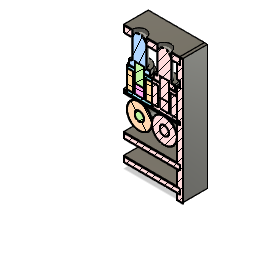
Braille Display Module CAD VA.1 (Autodesk Fusion 360 design; units mm, degrees)
Autodesk Fusion 360 part; units mm, degrees
note: some values were not read from the file. Chosen so that the rebuilt part matches the saved one: which bodies a step acts on; which face or edge a step refers to. Set by a fixed rule: which sketch regions a step uses.
sketch "Sketch1" plane through (0, 0, 0) normal (0, 0, 1) x (1, 0, 0)
  line L0 (-0.75, 2) -> (0.75, 2)
  line L1 (0.75, 2) -> (0.75, -2)
  line L2 (0.75, -2) -> (-0.75, -2)
  line L3 (-0.75, -2) -> (-0.75, 2)
  line L4 (0, 2) -> (0, -2)
  line L5 (0.75, -2) -> (2, -2)
  line L6 (2, -2) -> (2, -1.5)
  line L7 (2, -1.5) -> (0.75, -1.5)
  line L8 (0.75, -1.5) -> (0.75, -2)
  line L9 (0.75, -1.5) -> (-0.75, -1.5)
  line L10 (0.75, -1.5) -> (1, -1.5)
  line L11 (1, -1.5) -> (1, 2)
  line L12 (1, 2) -> (0.75, 2)
  line L13 (0.75, 2) -> (0.75, -1.5)
  line L14 (-0.75, -2) -> (-2, -2)
  line L15 (-2, -2) -> (-2, -1.5)
  line L16 (-2, -1.5) -> (-0.75, -1.5)
  line L17 (-0.75, -1.5) -> (-1, -1.5)
  line L18 (-1.25, 2.0006) -> (-0.75, 2)
  line L19 (-0.75, 2) -> (-0.75, -1.5)
  line L20 (-1, -1.5) -> (-1, 2)
  line L21 (1, 2) -> (2, 2)
  line L22 (2, 2) -> (2, 1.5)
  line L23 (2, 1.5) -> (1, 1.5)
  line L24 (1, 1.5) -> (1, 2)
  line L25 (2, -1.5) -> (2, 1.5)
  line L26 (-1, 2) -> (-2, 2)
  line L27 (-2, 2) -> (-2, 1.5)
  line L28 (-1, 1.5) -> (-1, 2)
  line L29 (-2, 1.5) -> (-1, 1.5)
  line L30 (-0.75, 0) -> (-0.75, 2.1)
  line L31 (-0.75, 2.1) -> (0.75, 2.1)
  line L32 (0.75, 2.1) -> (0.75, 0)
  line L33 (0, 2) -> (0, 2.1)
  line L34 (0.75, -1.5) -> (-0.75, -1.5)
  line L35 (-0.75, -1.5) -> (-0.75, 0)
  line L36 (-0.75, 0) -> (0.75, 0)
  line L37 (0.75, 0) -> (0.75, -1.5)
  line L38 (0.75, 2) -> (1.7, 2)
  line L39 (1.7, 2) -> (1.7, 2.1)
  line L40 (1.7, 2.1) -> (0.75, 2.1)
  line L41 (0.75, 2.1) -> (0.75, 2)
  line L42 (0.75, 2.1) -> (-0.75, 2.1)
  line L43 (-0.75, 2.1) -> (-0.75, 3)
  line L44 (-0.75, 3) -> (0.75, 3)
  line L45 (0.75, 3) -> (0.75, 2.1)
  line L46 (1.125, 2.1) -> (1.125, 3)
  line L47 (1.125, 3) -> (0.75, 3)
  line L48 (0, 3) -> (0, 4.8844)
  line L49 (0, 2.1) -> (0, 7.15)
  line L50 (1.125, 3) -> (1.125, 7.15)
  line L51 (1.125, 7.15) -> (-0.75, 7.15)
  line L52 (-0.75, 7.15) -> (-0.75, 3)
  line L53 (-1.125, 2.1) -> (-1.125, 3)
  line L54 (-1.125, 3) -> (-1.125, 7.15)
  line L55 (0.75, 7.15) -> (0.75, 3)
  line L56 (-0.75, 7.15) -> (-1.125, 7.15)
  line L57 (-0.75, 3) -> (-1.125, 3)
  line L58 (-0.75, 2.1) -> (-1.125, 2.1)
  line L59 (-1.125, 2.1) -> (-1.8, 2.1)
  line L60 (-1.8, 2.1) -> (-1.8, 2)
  line L61 (-1.125, 7.15) -> (-3, 7.15)
  line L62 (-3, 7.15) -> (-3, 6.15)
  line L63 (-3, 6.15) -> (-1.125, 6.15)
  line L64 (-1.125, 6.15) -> (-1.125, 7.15)
  line L65 (-3, 6.15) -> (-2, 6.15)
  line L66 (-2, 6.15) -> (-2, -2)
  line L67 (-2, -2) -> (-3, -2)
  line L68 (-3, -2) -> (-3, 6.15)
  line L69 (4.75, 2) -> (4.75, -1.5)
  line L70 (3.25, 2) -> (3.25, -1.5)
  line L71 (4.75, -2) -> (4.75, 2)
  line L72 (2, 1.5) -> (3, 1.5)
  line L73 (5, -1.5) -> (5, 2)
  line L74 (3, -1.5) -> (3, 2)
  line L75 (4, 2) -> (4, -2)
  line L76 (3.25, -2) -> (2, -2)
  line L77 (4.75, 2.1) -> (5.125, 2.1)
  line L78 (3.25, 2) -> (2.3, 2)
  line L79 (4.75, -2) -> (6, -2)
  line L80 (3.25, 0) -> (3.25, -1.5)
  line L81 (3.25, -1.5) -> (4.75, -1.5)
  line L82 (3.25, -1.5) -> (3, -1.5)
  line L83 (6, -2) -> (6, -1.5)
  line L84 (5.125, 2.1) -> (5.8, 2.1)
  line L85 (2.3, 2) -> (2.3, 2.1)
  line L86 (6, -1.5) -> (4.75, -1.5)
  line L87 (6, 6.15) -> (6, -2)
  line L88 (4.75, 3) -> (5.125, 3)
  line L89 (4, 3) -> (4, 4.8844)
  line L90 (3.25, 3) -> (3.25, 2.1)
  line L91 (7, -2) -> (7, 6.15)
  line L92 (3.25, -1.5) -> (4.75, -1.5)
  line L93 (4, 2.1) -> (4, 7.15)
  line L94 (3.25, 7.15) -> (3.25, 3)
  line L95 (6, 1.5) -> (5, 1.5)
  line L96 (4.75, -1.5) -> (4.75, 0)
  line L97 (2, -1.5) -> (3.25, -1.5)
  line L98 (4.75, -1.5) -> (5, -1.5)
  line L99 (3.25, 2) -> (3.25, -2)
  line L100 (5.125, 3) -> (5.125, 7.15)
  line L101 (4.75, 7.15) -> (4.75, 3)
  line L102 (4.75, 3) -> (3.25, 3)
  line L103 (2.875, 3) -> (2.875, 7.15)
  line L104 (2.3, 2.1) -> (3.25, 2.1)
  line L105 (5.125, 7.15) -> (7, 7.15)
  line L106 (3.25, -2) -> (4.75, -2)
  line L107 (3.25, -1.5) -> (3.25, -2)
  line L108 (4.75, 0) -> (3.25, 0)
  line L109 (3, 1.5) -> (3, 2)
  line L110 (7, 6.15) -> (6, 6.15)
  line L111 (2.875, 2.1) -> (2.875, 3)
  line L112 (6, -2) -> (7, -2)
  line L113 (3.25, 2.1) -> (3.25, 2)
  line L114 (7, 6.15) -> (5.125, 6.15)
  line L115 (4.75, 2) -> (3.25, 2)
  line L116 (5, 2) -> (6, 2)
  line L117 (4, 2) -> (4, 2.1)
  line L118 (3, 2) -> (2, 2)
  line L119 (5, 1.5) -> (5, 2)
  line L120 (7, 7.15) -> (7, 6.15)
  line L121 (4.75, 7.15) -> (5.125, 7.15)
  line L122 (4.75, 0) -> (4.75, 2.1)
  line L123 (4.75, 2.1) -> (3.25, 2.1)
  line L124 (5, 2) -> (4.75, 2)
  line L125 (3, 2) -> (3.25, 2)
  line L126 (2.875, 3) -> (3.25, 3)
  line L127 (5.125, 6.15) -> (5.125, 7.15)
  line L128 (5.8, 2.1) -> (5.8, 2)
  line L129 (2.875, 7.15) -> (4.75, 7.15)
  line L130 (6, 2) -> (6, 1.5)
  line L131 (4.75, 2.1) -> (4.75, 3)
  line L132 (3.25, 2.1) -> (4.75, 2.1)
  line L133 (3.25, 2.1) -> (3.25, 0)
  line L134 (5.125, 2.1) -> (5.125, 3)
  line L135 (1.125, 7.15) -> (2.875, 7.15)
  line L136 (2.875, 7.15) -> (2.875, 6.15)
  line L137 (2.875, 6.15) -> (1.125, 6.15)
  line L138 (1.125, 6.15) -> (1.125, 7.15)
  line L139 (5.125, 6.15) -> (-1.125, 6.15)
  line L140 (-1.125, 6.15) -> (-1.125, 7.15)
  line L141 (-1.125, 7.15) -> (5.125, 7.15)
  line L142 (5.125, 7.15) -> (5.125, 6.15)
  line L143 (-3, -2) -> (7, -2)
  line L144 (7, -2) -> (7, -2.25)
  line L145 (7, -2.25) -> (-3, -2.25)
  line L146 (-3, -2.25) -> (-3, -2)
  arc A0 (5.125, 6.15) -> (2.875, 6.15) centre (4, 6.0172) ccw
  arc A1 (1.125, 6.15) -> (-1.125, 6.15) centre (0, 6.0172) ccw
  line L147 (-2.5, 2.9) -> (-2.5, 3.9)
  line L148 (-2.5, 3.9) -> (-2, 3.9)
  line L149 (-2, 2.9) -> (-2.5, 2.9)
  line L150 (6, 2.9) -> (6.5, 2.9)
  line L151 (6.5, 2.9) -> (6.5, 3.9)
  line L152 (6.5, 3.9) -> (6, 3.9)
  line L153 (1.7, 2.1) -> (-1.8, 2.1)
  line L154 (-1.8, 2.1) -> (-1.8, 2.85)
  line L155 (-1.8, 2.85) -> (1.7, 2.85)
  line L156 (1.7, 2.85) -> (1.7, 2.1)
  line L157 (2.3, 2.1) -> (5.8, 2.1)
  line L158 (5.8, 2.1) -> (5.8, 2.85)
  line L159 (2.3, 2.85) -> (2.3, 2.1)
  line L160 (5.8, 2.85) -> (2.3, 2.85)
  line L161 (7, -1.75) -> (-3, -1.75)
  line L162 (6, -1.75) -> (6.5, -1.75)
  line L163 (6.5, -1.75) -> (6.5, -2.25)
  line L164 (6.5, -2.25) -> (6, -2.25)
  line L165 (6, -2.25) -> (6, -1.75)
  line L166 (-3, 7.15) -> (-2.5, 7.15)
  line L167 (-2.5, 7.15) -> (-2.5, 6.15)
  line L168 (-2.5, 6.15) -> (-3, 6.15)
  line L169 (-3, 6.15) -> (-3, 7.15)
  line L170 (7, 7.15) -> (6.5, 7.15)
  line L171 (6.5, 6.15) -> (7, 6.15)
  line L172 (7, 6.15) -> (7, 7.15)
  line L173 (6.5, 7.15) -> (6.5, 6.15)
  line L174 (-2, -2.25) -> (-2, -1.75)
  line L175 (-2, -1.75) -> (-2.5, -1.75)
  line L176 (-2.5, -2.25) -> (-2, -2.25)
  line L177 (-2.5, -1.75) -> (-2.5, -2.25)
  line L178 (-3, -2.25) -> (-2, -2.25)
  line L179 (-2, -2.25) -> (-2, -12.85)
  line L180 (-2, -12.85) -> (-3, -12.85)
  line L181 (-3, -12.85) -> (-3, -2.25)
  line L182 (7, -2.25) -> (6, -2.25)
  line L183 (6, -2.25) -> (6, -12.85)
  line L184 (6, -12.85) -> (7, -12.85)
  line L185 (7, -12.85) -> (7, -2.25)
  line L186 (-2.5, -7.75) -> (6.5, -7.75)
  line L187 (6.5, -7.75) -> (6.5, -8.55)
  line L188 (6.5, -8.55) -> (-2.5, -8.55)
  line L189 (-2.5, -8.55) -> (-2.5, -7.75)
  line L190 (-2.5, -11.05) -> (6.5, -11.05)
  line L191 (6.5, -11.05) -> (6.5, -11.85)
  line L192 (6.5, -11.85) -> (-2.5, -11.85)
  line L193 (-2.5, -11.85) -> (-2.5, -11.05)
  line L194 (-2, -6.25) -> (6, -6.25)
  line L195 (2, -2.25) -> (2, -6.25)
  line L196 (2, -4.25) -> (6, -4.25) construction
  circle A2 centre (0, -4.25) radius 0.75
  circle A3 centre (4, -4.25) radius 0.75
  circle A4 centre (0, -4.25) radius 2
  circle A5 centre (4, -4.25) radius 2
  point P0 (4, 0)
  dimension "d4" = 0.25
  dimension "d7" = 0.5
  dimension "d8" = 4
  dimension "d9" = 0.5
  dimension "d21" = 1.5
  dimension "d22" = 1.5
  dimension "d27" = 0.1
  dimension "d31" = 1
  dimension "d32" = 1
  dimension "d37" = 0.25
  dimension "d57" = 1
  dimension "d60" = 0.5
  dimension "d63" = 1.8
  dimension "d64" = 0.75
  dimension "d68" = 2.25
  dimension "d69" = 3
  dimension "d70" = 3
  dimension "d72" = 2.25
  dimension "d73" = 0.25
  dimension "d74" = 0.5
  dimension "d76" = 0.5
  dimension "d77" = 0.5
  dimension "d78" = 0.8
  dimension "d79" = 0.8
  dimension "d80" = 0.5
  dimension "d81" = 0.5
  dimension "d82" = 2.5
  dimension "d85" = 1.5
  dimension "d97" = 4
  dimension "d100" = 1.5
  dimension "d101" = 1.5
  dimension "d104" = 3.5
  dimension "d105" = 20
  constraint horizontal L0
  constraint vertical L1
  constraint horizontal L2
  constraint vertical L3
  constraint midpoint L0 L4.start
  constraint midpoint L2 L4.end
  constraint coincident origin L4
  constraint horizontal L5
  constraint vertical L6
  constraint horizontal L7
  constraint vertical L8
  constraint coincident L3 L9.end
  constraint perpendicular L3 L9
  constraint horizontal L10
  constraint vertical L11
  constraint horizontal L12
  constraint vertical L13
  constraint coincident L0.end L1.start
  constraint symmetric L1.end L4 L2.end
  constraint symmetric L4 L5.end L14.end
  constraint symmetric L4 L6.end L15.end
  constraint symmetric L4 L7.end L9.end
  constraint symmetric L4 L10.end L17.end
  constraint symmetric L4 L11.end L20.end
  constraint symmetric L4 L0.end L0.start
  constraint horizontal L21
  constraint vertical L22
  constraint horizontal L23
  constraint vertical L24
  constraint vertical L25
  constraint symmetric L4 L21.end L26.end
  constraint symmetric L4 L22.end L27.end
  constraint symmetric L4 L23.end L28.start
  constraint vertical L30
  constraint horizontal L31
  constraint vertical L32
  constraint perpendicular L31 L33
  constraint coincident L31 L33.end
  constraint horizontal L34
  constraint vertical L35
  constraint horizontal L36
  constraint vertical L37
  constraint coincident L19 L30.start
  constraint coincident L3 L30.start
  constraint coincident L1 L32.end
  constraint coincident L32.end L36.end
  constraint coincident L30.start L36
  constraint coincident origin L36
  constraint horizontal L38
  constraint vertical L39
  constraint horizontal L40
  constraint vertical L41
  constraint coincident L32 L0.end
  constraint coincident L21 L38.end
  constraint horizontal L42
  constraint vertical L43
  constraint horizontal L44
  constraint vertical L45
  constraint coincident L30.end L31.start
  constraint coincident L31.end L32.start
  constraint coincident L40 L46.start
  constraint perpendicular L40 L46
  constraint horizontal L47
  constraint midpoint L44 L48.start
  constraint perpendicular L44 L48
  constraint perpendicular L43 L51
  constraint perpendicular L44 L52
  constraint symmetric L46.end L48 L53.end
  constraint symmetric L43.end L48 L44.end
  constraint symmetric L46.start L48 L53.start
  constraint symmetric L48 L50.end L54.end
  constraint symmetric L48 L51.end L55.start
  constraint perpendicular L43 L59
  constraint coincident L26 L60.end
  constraint perpendicular L26 L60
  constraint horizontal L61
  constraint vertical L62
  constraint horizontal L63
  constraint vertical L64
  constraint horizontal L65
  constraint vertical L66
  constraint horizontal L67
  constraint vertical L68
  constraint symmetric origin L25 P0
  constraint symmetric L0.start L25 L69.start
  constraint symmetric L0.end L25 L70.start
  constraint symmetric L1.end L25 L76.start
  constraint symmetric L2.end L25 L71.start
  constraint symmetric L4.start L25 L75.start
  constraint symmetric L4.end L25 L75.end
  constraint symmetric L32.end L25 L80.start
  constraint symmetric L5.end L25 L6.start
  constraint symmetric L6.end L25 L7.start
  constraint symmetric L7.end L25 L70.end
  constraint symmetric L9.end L25 L69.end
  constraint symmetric L10.end L25 L74.start
  constraint symmetric L11.end L25 L74.end
  constraint symmetric L14.end L25 L79.end
  constraint symmetric L15.end L25 L83.end
  constraint symmetric L17.end L25 L73.start
  constraint symmetric L20.end L25 L73.end
  constraint symmetric L21.end L25 L22.start
  constraint symmetric L22.end L25 L23.start
  constraint symmetric L23.end L25 L72.end
  constraint symmetric L25 L20.end L73.end
  constraint symmetric L25 L26.end L116.end
  constraint symmetric L25 L27.end L95.start
  constraint symmetric L25 L28.start L95.end
  constraint symmetric L25 L30.start L96.end
  constraint symmetric L25 L30.end L77.start
  constraint symmetric L25 L31.end L90.end
  constraint symmetric L25 L33.end L93.start
  constraint symmetric L25 L9.end L69.end
  constraint symmetric L25 L32.end L80.start
  constraint symmetric L25 L0.end L70.start
  constraint symmetric L25 L38.end L78.end
  constraint symmetric L25 L39.end L85.end
  constraint symmetric L25 L43.end L88.start
  constraint symmetric L25 L44.end L90.start
  constraint symmetric L25 L46.start L111.start
  constraint symmetric L25 L46.end L103.start
  constraint symmetric L25 L48.start L89.start
  constraint symmetric L25 L48.end L89.end
  constraint symmetric L25 L49.end L93.end
  constraint symmetric L25 L50.end L103.end
  constraint symmetric L25 L51.end L101.start
  constraint symmetric L25 L53.end L88.end
  constraint symmetric L25 L53.start L77.end
  constraint symmetric L25 L54.end L100.end
  constraint symmetric L25 L55.start L94.start
  constraint symmetric L25 L59.end L84.end
  constraint symmetric L25 L60.end L128.end
  constraint symmetric L25 L61.end L105.end
  constraint symmetric L25 L62.end L91.end
  constraint symmetric L25 L63.end L114.end
  constraint symmetric L25 L65.end L87.start
  constraint symmetric L25 L67.end L91.start
  constraint horizontal L135
  constraint vertical L136
  constraint horizontal L137
  constraint vertical L138
  constraint coincident L103 L136.end
  constraint horizontal L139
  constraint vertical L140
  constraint horizontal L141
  constraint vertical L142
  constraint horizontal L143
  constraint vertical L144
  constraint horizontal L145
  constraint vertical L146
  constraint coincident L91.start L112.end
  constraint coincident L89.end A0
  constraint tangent L141 A0
  constraint symmetric L25 L114.end L63.end
  constraint symmetric L25 L136.end L137.end
  constraint symmetric L25 A0 A1
  constraint coincident L139 L114.end
  constraint vertical L100
  constraint coincident L114.end L127.start
  constraint coincident L136.end L137.start
  constraint perpendicular L26 L147
  constraint coincident L66 L148.end
  constraint perpendicular L66 L148
  constraint coincident L66 L149.start
  constraint horizontal L149
  constraint horizontal L26
  constraint coincident L26.end L27.start
  constraint symmetric L25 L147.start L150.end
  constraint symmetric L25 L147.end L151.end
  constraint symmetric L25 L148.end L152.end
  constraint symmetric L25 L149.start L150.start
  constraint horizontal L153
  constraint vertical L154
  constraint horizontal L155
  constraint vertical L156
  constraint coincident L59.end L60.start
  constraint symmetric L25 L154.end L158.end
  constraint symmetric L25 L155.end L159.start
  constraint coincident L139 L137.end
  constraint coincident L91 L161.start
  constraint coincident L68 L161.end
  constraint perpendicular L68 L161
  constraint horizontal L162
  constraint vertical L163
  constraint horizontal L164
  constraint vertical L165
  constraint coincident L145 L163.end
  constraint midpoint L83 L162.start
  constraint horizontal L166
  constraint vertical L167
  constraint horizontal L168
  constraint vertical L169
  constraint midpoint L65 L167.end
  constraint symmetric L25 L162.start L174.end
  constraint symmetric L25 L162.end L175.end
  constraint symmetric L25 L163.end L176.start
  constraint symmetric L25 L164.end L174.start
  constraint symmetric L25 L166.end L170.end
  constraint symmetric L25 L167.end L171.start
  constraint horizontal L178
  constraint vertical L179
  constraint horizontal L180
  constraint vertical L181
  constraint coincident L174.start L176.end
  constraint horizontal L182
  constraint vertical L183
  constraint horizontal L184
  constraint vertical L185
  constraint coincident L164.end L165.start
  constraint equal L179 L183
  constraint horizontal L186
  constraint vertical L187
  constraint horizontal L188
  constraint vertical L189
  constraint horizontal L190
  constraint vertical L191
  constraint horizontal L192
  constraint vertical L193
  constraint coincident L179 L194.start
  constraint coincident L183 L194.end
  constraint perpendicular L183 L194
  constraint coincident L49.end L141
  constraint midpoint L145 L195.start
  constraint midpoint L194 L195.end
  constraint midpoint L195 L196.start
  constraint coincident L183 L196.end
  constraint perpendicular L183 L196
  constraint concentric A2 A4
  constraint tangent L194 A4
  constraint concentric A3 A5
  constraint tangent L194 A5
  constraint tangent L195 A5
  constraint tangent L195 A4
  constraint tangent L145 A4
  constraint tangent L145 A5
  measures "d4" distance of L11.end L0.end
  measures "d7" distance of L5 L7
  measures "d8" distance of L5.end L14.end
  measures "d9" distance of L21 L23
  measures "d21" distance of L30.end L31.end
  measures "d22" distance of L9 L36
  measures "d27" distance of L38.end L39.end
  measures "d31" distance of L66 L68
  measures "d32" distance of L61 L63
  measures "d37" distance of L112 L145
  measures "d57" distance of L147.start L147.end
  measures "d60" distance of L66 L147
  measures "d63" vertical distance of L59.end L147.end
  measures "d64" distance of L153 L155
  measures "d68" distance of L46 L53
  measures "d69" distance of L36 L44
  measures "d70" distance of L16 L29
  measures "d72" distance of L65 L148
  measures "d73" distance of L143 L161
  measures "d74" distance of L163 L165
  measures "d76" distance of L179 L189
  measures "d77" distance of L183 L187
  measures "d78" distance of L186 L188
  measures "d79" distance of L190 L192
  measures "d80" distance of L183 L191
  measures "d81" distance of L179 L193
  measures "d82" distance of L188 L190
  measures "d85" distance of L186 L194
  measures "d97" distance of L145 L194
  measures "d100" diameter of A2
  measures "d101" diameter of A3
  measures "d104" distance of L154 L156
  measures "d105" distance of L61.end L180
revolve "Revolve1" add sketch "Sketch1" angle 360 about axis through (0, 1.75, 0) along (0, 1, 0) contours L1 L7 L10 L11 L12 L13 L24 L32 L37 L38 | L11 L21 L22 L23 L24 L38 | L1 L4 L8 L9 L34 L161 | L1 L6 L7 L8 L10 L161 | L1 L2 L4 L8 L143 L161 | L1 L5 L6 L8 L143 L161 makes body 1
revolve "Revolve2" add sketch "Sketch1" angle 360 about axis through (0, 1.75, 0) along (0, 1, 0) separate body contours L1 L4 L9 L13 L34 L36 L37 makes body 2
revolve "Revolve3" add sketch "Sketch1" angle 360 about axis through (0, 1.75, 0) along (0, 1, 0) separate body contours L7 L11 L23 L25 makes body 3
revolve "Revolve4" add sketch "Sketch1" angle 360 about axis through (0, 2, 0) along (0, 1, 0) separate body contours L0 L31 L32 L33 L41 L42 L153 | L0 L1 L4 L13 L32 L36 | L31 L42 L45 L49 L153 L155 | L44 L45 L49 L155 makes body 4
revolve "Revolve5" add sketch "Sketch1" angle 360 about axis through (0, 2.1, 0) along (0, 1, 0) separate body contours L40 L45 L46 L153 L155 | L40 L46 L153 L155 L156 | L45 L46 L47 L155 | L44 L48 L49 L55 L139 | L47 L50 L55 L139 | L49 L55 L139 A1 | L55 L139 A1 makes body 5
revolve "Revolve7" add sketch "Sketch1" angle 360 about axis through (0, 2, 0) along (0, -1, 0) separate body contours L12 L21 L32 L38 L39 L40 L41 L153 makes body 6
extrude "Extrude1" add sketch "Sketch1" along normal blind 12 and the other way blind 4 separate body contours L15 L27 L63 L65 L66 L68 L147 L148 L149 L161 L168 L175 | L67 L68 L143 L161 L177 | L67 L143 L145 L146 L177 L178 | L145 L176 L178 L179 L180 L181 L186 L188 L189 L190 L192 L193 | L61 L62 L63 L65 L166 L167 L168 L169 | L83 L87 L91 L110 L114 L130 L150 L151 L152 L161 L162 L171 | L145 L164 L182 L183 L184 L185 L186 L187 L188 L190 L191 L192 | L91 L112 L143 L161 L163 | L112 L143 L144 L145 L163 L182 | L105 L110 L114 L120 L170 L171 L172 L173 makes body 7 at (-3, -6.1833, 6.6667) makes body 8 at (7, 0.4833, 1.3333)
extrude "Extrude4" add sketch "Sketch1" along normal blind 12 and the other way blind 4 separate body contours L2 L3 L4 L143 L161 | L3 L14 L15 L66 L143 L161 L174 | L1 L2 L4 L8 L143 L161 | L15 L66 L67 L143 L161 L174 L175 L177 | L52 L139 A1 | L49 L52 L139 A1 | L1 L5 L6 L8 L143 L161 | L52 L54 L56 L64 L140 L141 A1 | L51 L52 L141 A1 | L49 L55 L139 A1 | L54 L61 L63 L64 L65 L140 L167 | L6 L76 L99 L107 L143 L161 | L55 L139 A1 | L51 L55 L141 A1 | L75 L99 L106 L107 L143 L161 | L50 L51 L55 L138 L141 A1 | L50 L103 L135 L136 L137 L138 L139 L141 | L71 L75 L106 L143 L161 | L94 L139 A0 | L94 L103 L129 L136 L141 A0 | L71 L79 L83 L87 L143 L161 L165 | L93 L94 L139 A0 | L94 L129 L141 A0 | L179 L183 L186 L188 | L179 L186 L188 L189 | L83 L87 L112 L143 L161 L162 L163 L165 | L93 L101 L139 A0 | L101 L129 L141 A0 | L183 L186 L187 L188 | L101 L139 A0 | L100 L101 L121 L127 L141 L142 A0 | L179 L190 L192 L193 | L179 L183 L190 L192 | L100 L105 L110 L114 L127 L142 L173 | L183 L190 L191 L192 makes body 9 at (3.5, -2, 6.6667) makes body 10 at (0.5, -7.75, 6.6667) makes body 11 at (3.5, 6.15, 1.3333) makes body 12 at (0.5, -11.05, 6.6667)
extrude "Extrude5" add sketch "Sketch1" along normal blind 12 and the other way blind 4 separate body contours L2 L5 L14 L76 L79 L106 L143 L145 L165 L174 | L67 L143 L145 L174 L176 L177 L178 | L112 L143 L145 L163 L164 L165 L182 makes body 13
revolve "Revolve6" cut sketch "Sketch1" angle 360 about axis through (0, 3, 0) along (0, 1, 0) contours L1 L2 L4 L8 L143 L161 | L44 L48 L49 L55 L139 | L1 L5 L6 L8 L143 L161 | L47 L50 L55 L139 | L49 L55 L139 A1 | L55 L139 A1 | L51 L55 L141 A1 | L50 L51 L55 L138 L141 A1 bodies 9 11
pattern_linear "R-Pattern2" count 2 spacing 4 along (1, 0, 0) count 3 spacing 4 along (0, 0, 1) of "Revolve6"
pattern_linear "R-Pattern1" count 2 spacing 4 along (1, 0, 0) count 3 spacing 4 along (0, 0, 1) of bodies 5 3 1 4 2 6 makes body 14 at (5.5759, -2, 0.0994) makes body 15 at (1.5759, -2, 4.0994) makes body 16 at (5.5759, -2, 4.0994) makes body 17 at (1.5759, -2, 8.0994) makes body 18 at (5.5759, -2, 8.0994) makes body 19 at (4.7491, -0.5, 0.0374) makes body 20 at (0.7491, -0.5, 4.0374) makes body 21 at (4.7491, -0.5, 4.0374) makes body 22 at (0.7491, -0.5, 8.0374) makes body 23 at (4.7491, -0.5, 8.0374) makes body 24 at (5.9901, -0.5, 0.1991) makes body 25 at (1.9901, -0.5, 4.1991) makes body 26 at (5.9901, -0.5, 4.1991) makes body 27 at (1.9901, -0.5, 8.1991) makes body 28 at (5.9901, -0.5, 8.1991) makes body 29 at (4.7491, 1.3333, 0.0374) makes body 30 at (0.7491, 1.3333, 4.0374) makes body 31 at (4.7491, 1.3333, 4.0374) makes body 32 at (-0.7463, 1.3333, 8.0747) makes body 33 at (3.2537, 1.3333, 8.0747) makes body 34 at (5.1236, 4.05, 0.0561) makes body 35 at (1.1236, 4.05, 4.0561) makes body 36 at (5.1236, 4.05, 4.0561) makes body 37 at (1.1236, 4.05, 8.0561) makes body 38 at (5.1236, 4.05, 8.0561) makes body 39 at (5.6916, 2.0667, -0.1693) makes body 40 at (1.6979, 2.0333, 3.9153) makes body 41 at (5.6916, 2.0667, 3.8307) makes body 42 at (1.6979, 2.0333, 7.9153) makes body 43 at (5.6916, 2.0667, 7.8307)
extrude "Extrude6" cut 2 faces at (1.9044, -1.75, 6.1628) (1.9044, -1.75, 2.1628) along direction (0, -1, 0) blind 1 on bodies 9 bodies 9
extrude "Extrude7" add sketch "Sketch1" along normal blind 12 and the other way blind 4 separate body contours A5 | A2 makes body 44 at (0.7491, -4.2874, 8) makes body 45 at (5.9901, -4.4491, 1.3333)
extrude "Extrude8" add sketch "Sketch1" along normal blind 12 and the other way blind 4 separate body contours A4 | A3 makes body 46 at (1.9901, -4.4491, 1.3333) makes body 47 at (4.7491, -4.2874, 8)
copy_body "Body->Comp1" bodies 1 removing the originals makes body 48 in component "Magnet Core"
copy_body "Body->Comp2" bodies 2 removing the originals makes body 49 in component "Magnet"
copy_body "Body->Comp3" bodies 3 removing the originals makes body 50 in component "Coil"
copy_body "Body->Comp4" bodies 4 removing the originals makes body 51 in component "Pin"
copy_body "Body->Comp5" bodies 5 removing the originals makes body 52 in component "PinHat"
copy_body "Body->Comp6" bodies 6 removing the originals makes body 53 in component "Felt"
copy_body "Body->Comp7" bodies 46 removing the originals makes body 54 in component "EnableCoil1"
copy_body "Body->Comp8" bodies 44 removing the originals makes body 55 in component "EnableCore1"
component "Magnet Core" placed x (1, 0, 0) y (0, 1, 0) z (0, 0, 1) at (0, 0, 0)
component "Magnet" placed x (1, 0, 0) y (0, 1, 0) z (0, 0, 1) at (0, 0, 0)
component "Coil" placed x (1, 0, 0) y (0, 1, 0) z (0, 0, 1) at (0, 0, 0)
component "Pin" placed x (1, 0, 0) y (0, 1, 0) z (0, 0, 1) at (0, 0, 0)
component "PinHat" placed x (1, 0, 0) y (0, 1, 0) z (0, 0, 1) at (0, 0, 0)
component "Felt" placed x (1, 0, 0) y (0, 1, 0) z (0, 0, 1) at (0, 0, 0)
component "EnableCoil1" placed x (1, 0, 0) y (0, 1, 0) z (0, 0, 1) at (0, 0, 0)
component "EnableCore1" placed x (1, 0, 0) y (0, 1, 0) z (0, 0, 1) at (0, 0, 0)
hidden bodies 7
equation "d42 = 10.00 mm + 2 mm"
equation "d44 = 2.00 mm + 2 mm"
equation "d72 = d64 + 1.5 mm"
equation "d74 = d60"
equation "d76 = d60"
equation "d77 = d60"
equation "d79 = d78"
equation "d80 = d60"
equation "d81 = d60"
named bodies: "Magnet Core", "Magnet", "Coil", "Pin", "PinHat", "Magnet Core (1)", "Magnet Core (2)", "Magnet Core (3)", "Magnet Core (4)", "Magnet Core (5)", "Magnet (1)", "Magnet (2)", "Magnet (3)", "Magnet (4)", "Magnet (5)", "Coil (1)", "Coil (2)", "Coil (3)", "Coil (4)", "Coil (5)", "Pin (1)", "Pin (2)", "Pin (3)", "Pin (4)", "Pin (5)", "PinHat (1)", "PinHat (2)", "PinHat (3)", "PinHat (4)", "PinHat (5)", "Left Side", "Felt", "Felt (1)", "Felt (2)", "Felt (3)", "Felt (4)", "Felt (5)", "Right Side", "Middle Plate", "Top PCB", "Top Plate", "Bottom PCB", "Metal Plate", "EnableCore1", "EnableCoil2", "EnableCoil1", "EnableCore2"
